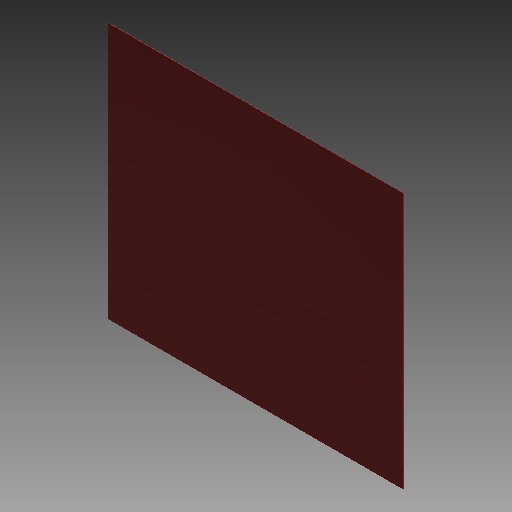
# Autodesk Inventor part: OSHW_LOGO_8MILX0150-NT
Saved by Autodesk Inventor 2018.2 (Build 222227000, 227)
## iProperties
Part Number: OSHW_LOGO_8MILX0150-NT
Material: Generic
Document SubType Name: Modeling
Designer: autocad
Appearance: OSHW_8X150_NOTEXT, OSHW_LOGO_8MILX0150-NT
Author: autocad
Autodesk Inventor part; units mm, degrees
ref_plane "YZ Plane" through (0, 0, 0) normal (1, 0, 0) x (0, 1, 0)
ref_plane "XZ Plane" through (0, 0, 0) normal (0, 1, 0) x (-1, 0, 0)
ref_plane "XY Plane" through (0, 0, 0) normal (0, 0, 1) x (1, 0, 0)
sketch "OSHW_8X150_NOTEXT, OSHW_LOGO_8MILX0150-NT_73" plane through (0, 0, 0) normal (0, 0, 1) x (1, 0, 0)
  line L0 (4.2672, 0.0508) -> (-0.0018, 0.0508)
  line L1 (-0.0018, 0.0508) -> (-0.0018, 3.7592)
  line L2 (-0.0018, 3.7592) -> (4.2672, 3.7592)
  line L3 (4.2672, 3.7592) -> (4.2672, 0.0508)
  constraints: 8 end point
extrude "Extrusion1" add sketch "OSHW_8X150_NOTEXT, OSHW_LOGO_8MILX0150-NT_73" along normal blind 0.01
body "Solid1"
